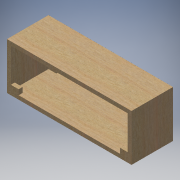
# Autodesk Inventor part: cabinet
Saved by Autodesk Inventor 2016 (Build 200138000, 138)
## iProperties
Created: 2015-10-14
Part Number: cabinet
Material: Pine, Radiata
Document SubType Name: Modeling
Designer: jeremyhale
Density: 0.48 g/cm^3
Appearance: Pine - Coarse
Author: jeremyhale
Autodesk Inventor part; units mm, degrees
ref_plane "YZ Plane" through (0, 0, 0) normal (1, 0, 0) x (0, 1, 0)
ref_plane "XZ Plane" through (0, 0, 0) normal (0, 1, 0) x (-1, 0, 0)
ref_plane "XY Plane" through (0, 0, 0) normal (0, 0, 1) x (1, 0, 0)
sketch "Sketch1" plane through (0, 0, 0) normal (0, 1, 0) x (-1, 0, 0)
  line L0 (-304.8, 101.6) -> (304.8, 101.6)
  line L1 (304.8, 101.6) -> (304.8, -101.6)
  line L2 (304.8, -101.6) -> (-304.8, -101.6)
  line L3 (-304.8, -101.6) -> (-304.8, 101.6)
  line L4 (-304.8, 101.6) -> (304.8, -101.6) construction
  line L5 (304.8, 101.6) -> (-304.8, -101.6) construction
  point P0 (0, 0)
  dimension "length" = 609.6
  dimension "width" = 203.2
  constraints: 12 end point, 2 midpoint, 2 parallel, 1 horizontal, 1 perpendicular
  measures "length" distance of L1.end L2.end
  measures "width" distance of L0.end L1.end
extrude "Extrusion1" add sketch "Sketch1" along normal blind 19.05
sketch "Sketch2" plane through (0, 19.05, 0) normal (0, 1, 0) x (1, 0, 0)
  line L0 (-304.8, -101.6) -> (304.8, -101.6) projected
  line L1 (304.8, 101.6) -> (-304.8, 101.6) projected
  line L2 (-304.8, -101.6) -> (-304.8, 101.6)
  line L3 (-304.8, 101.6) -> (-285.75, 101.6)
  line L4 (-285.75, 101.6) -> (-285.75, -101.6)
  line L5 (-285.75, -101.6) -> (-304.8, -101.6)
  point P0 (0, 0)
  dimension "d4" = 19.05
  constraints: 8 end point, 2 parallel, 1 perpendicular, 1 vertical
  measures "d4" distance of L1.end L3.end
extrude "Extrusion2" add sketch "Sketch2" along normal blind 190.5
mirror "Mirror2" about plane through (0, 0, 0) normal (1, 0, 0) of "Extrusion2"
sketch "Sketch3" plane through (0, 19.05, 0) normal (0, 1, 0) x (1, 0, 0)
  line L0 (-285.75, -101.6) -> (-247.65, -101.6)
  line L1 (-247.65, -101.6) -> (-247.65, -82.55)
  line L2 (-247.65, -82.55) -> (-285.75, -82.55)
  line L3 (-285.75, -82.55) -> (-285.75, -101.6)
  line L4 (-285.75, -101.6) -> (285.75, -101.6)
  line L5 (285.75, -101.6) -> (247.65, -101.6)
  line L6 (247.65, -101.6) -> (247.65, -82.55)
  line L7 (247.65, -82.55) -> (285.75, -82.55)
  line L8 (285.75, -82.55) -> (285.75, -101.6)
  point P0 (0, 0)
  dimension "d7" = 19.05
  dimension "d8" = 19.05
  dimension "d12" = 38.1
  dimension "d14" = 38.1
  constraints: 18 end point, 4 parallel, 2 horizontal, 2 perpendicular
  measures "d7" distance of L0.end L1.end
  measures "d8" distance of L5.end L6.end
  measures "d12" distance between parallel lines of L8 L6
  measures "d14" distance between parallel lines of L1 L3
extrude "Extrusion3" add sketch "Sketch3" along normal blind 25.4
mirror "Mirror3" about plane through (0, 0, 0) normal (0, 0, 1) of "Extrusion3"
sketch "Sketch5" plane through (0, 209.55, 0) normal (0, 1, 0) x (1, 0, 0)
  line L0 (304.8, -101.6) -> (-304.8, -101.6) projected
  line L1 (304.8, 101.6) -> (304.8, -101.6) projected
  line L2 (-304.8, -101.6) -> (304.8, -101.6)
  line L3 (304.8, -101.6) -> (304.8, 101.6)
  line L4 (304.8, 101.6) -> (-304.8, 101.6)
  line L5 (-304.8, 101.6) -> (-304.8, -101.6)
  point P0 (0, 0)
  constraints: 8 end point, 2 parallel, 1 horizontal, 1 perpendicular
extrude "Extrusion4" add sketch "Sketch5" along normal blind 19.05
equation "\"d4\" = thickness"
equation "\"d7\" = thickness"
equation "\"d8\" = thickness"
equation "\"d14\" = d12"
equation "\"d15\" = thickness"
equation "\"thickness\" = 19.05"
body "Solid1"
